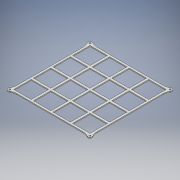
# Autodesk Inventor part: b-base
Saved by Autodesk Inventor 2017 (Build 210142000, 142)
## iProperties
Created: 2019-02-09
Part Number: b-base
Material: Generic
Document SubType Name: Modeling
Designer: felix
Density: 1 g/cm^3
Appearance: Default
Author: felix
Autodesk Inventor part; units mm, degrees
ref_plane "YZ Plane" through (0, 0, 0) normal (1, 0, 0) x (0, 1, 0)
ref_plane "XZ Plane" through (0, 0, 0) normal (0, 1, 0) x (-1, 0, 0)
ref_plane "XY Plane" through (0, 0, 0) normal (0, 0, 1) x (1, 0, 0)
sketch "Sketch1" plane through (0, 0, 0) normal (0, 0, 1) x (1, 0, 0)
  line L0 (-23.6233, -6.7963) -> (65.3767, -6.7963)
  line L1 (65.3767, -6.7963) -> (65.3767, 82.2037)
  line L2 (65.3767, 82.2037) -> (-23.6233, 82.2037)
  line L3 (-23.6233, 82.2037) -> (-23.6233, -6.7963)
  line L4 (-23.6233, 93.2037) -> (65.3767, 93.2037)
  line L5 (65.3767, 93.2037) -> (65.3767, 182.2037)
  line L6 (65.3767, 182.2037) -> (-23.6233, 182.2037)
  line L7 (-23.6233, 182.2037) -> (-23.6233, 93.2037)
  line L8 (-23.6233, 193.2037) -> (65.3767, 193.2037)
  line L9 (65.3767, 193.2037) -> (65.3767, 282.2037)
  line L10 (65.3767, 282.2037) -> (-23.6233, 282.2037)
  line L11 (-23.6233, 282.2037) -> (-23.6233, 193.2037)
  line L12 (-23.6233, 293.2037) -> (65.3767, 293.2037)
  line L13 (65.3767, 293.2037) -> (65.3767, 382.2037)
  line L14 (65.3767, 382.2037) -> (-23.6233, 382.2037)
  line L15 (-23.6233, 382.2037) -> (-23.6233, 293.2037)
  line L16 (76.3767, -6.7963) -> (165.3767, -6.7963)
  line L17 (165.3767, -6.7963) -> (165.3767, 82.2037)
  line L18 (165.3767, 82.2037) -> (76.3767, 82.2037)
  line L19 (76.3767, 82.2037) -> (76.3767, -6.7963)
  line L20 (76.3767, 93.2037) -> (165.3767, 93.2037)
  line L21 (165.3767, 93.2037) -> (165.3767, 182.2037)
  line L22 (165.3767, 182.2037) -> (76.3767, 182.2037)
  line L23 (76.3767, 182.2037) -> (76.3767, 93.2037)
  line L24 (76.3767, 193.2037) -> (165.3767, 193.2037)
  line L25 (165.3767, 193.2037) -> (165.3767, 282.2037)
  line L26 (165.3767, 282.2037) -> (76.3767, 282.2037)
  line L27 (76.3767, 282.2037) -> (76.3767, 193.2037)
  line L28 (76.3767, 293.2037) -> (165.3767, 293.2037)
  line L29 (165.3767, 293.2037) -> (165.3767, 382.2037)
  line L30 (165.3767, 382.2037) -> (76.3767, 382.2037)
  line L31 (76.3767, 382.2037) -> (76.3767, 293.2037)
  line L32 (176.3767, -6.7963) -> (265.3767, -6.7963)
  line L33 (265.3767, -6.7963) -> (265.3767, 82.2037)
  line L34 (265.3767, 82.2037) -> (176.3767, 82.2037)
  line L35 (176.3767, 82.2037) -> (176.3767, -6.7963)
  line L36 (176.3767, 93.2037) -> (265.3767, 93.2037)
  line L37 (265.3767, 93.2037) -> (265.3767, 182.2037)
  line L38 (265.3767, 182.2037) -> (176.3767, 182.2037)
  line L39 (176.3767, 182.2037) -> (176.3767, 93.2037)
  line L40 (176.3767, 193.2037) -> (265.3767, 193.2037)
  line L41 (265.3767, 193.2037) -> (265.3767, 282.2037)
  line L42 (265.3767, 282.2037) -> (176.3767, 282.2037)
  line L43 (176.3767, 282.2037) -> (176.3767, 193.2037)
  line L44 (176.3767, 293.2037) -> (265.3767, 293.2037)
  line L45 (265.3767, 293.2037) -> (265.3767, 382.2037)
  line L46 (265.3767, 382.2037) -> (176.3767, 382.2037)
  line L47 (176.3767, 382.2037) -> (176.3767, 293.2037)
  line L48 (276.3767, -6.7963) -> (365.3767, -6.7963)
  line L49 (365.3767, -6.7963) -> (365.3767, 82.2037)
  line L50 (365.3767, 82.2037) -> (276.3767, 82.2037)
  line L51 (276.3767, 82.2037) -> (276.3767, -6.7963)
  line L52 (276.3767, 93.2037) -> (365.3767, 93.2037)
  line L53 (365.3767, 93.2037) -> (365.3767, 182.2037)
  line L54 (365.3767, 182.2037) -> (276.3767, 182.2037)
  line L55 (276.3767, 182.2037) -> (276.3767, 93.2037)
  line L56 (276.3767, 193.2037) -> (365.3767, 193.2037)
  line L57 (365.3767, 193.2037) -> (365.3767, 282.2037)
  line L58 (365.3767, 282.2037) -> (276.3767, 282.2037)
  line L59 (276.3767, 282.2037) -> (276.3767, 193.2037)
  line L60 (276.3767, 293.2037) -> (365.3767, 293.2037)
  line L61 (365.3767, 293.2037) -> (365.3767, 382.2037)
  line L62 (365.3767, 382.2037) -> (276.3767, 382.2037)
  line L63 (276.3767, 382.2037) -> (276.3767, 293.2037)
  circle A0 centre (-33.6233, -16.7963) radius 4
  arc A1 (-42.1947, -11.6455) -> (-33.6233, 19.2592) centre (-93.6233, 19.2592) ccw
  arc A2 (2.4322, -16.7963) -> (-28.4725, -25.3677) centre (2.4322, -76.7963) ccw
  arc A3 (-42.1947, -11.6455) -> (-28.4725, -25.3677) centre (-33.6233, -16.7963) ccw
  arc A4 (375.3767, 19.2592) -> (383.9481, -11.6455) centre (435.3767, 19.2592) ccw
  circle A5 centre (375.3767, -16.7963) radius 4
  arc A6 (370.2259, -25.3677) -> (383.9481, -11.6455) centre (375.3767, -16.7963) ccw
  arc A7 (370.2259, -25.3677) -> (339.3212, -16.7963) centre (339.3212, -76.7963) ccw
  arc A8 (339.3212, 392.2037) -> (370.2259, 400.7751) centre (339.3212, 452.2037) ccw
  circle A9 centre (375.3767, 392.2037) radius 4
  arc A10 (383.9481, 387.0529) -> (370.2259, 400.7751) centre (375.3767, 392.2037) ccw
  arc A11 (383.9481, 387.0529) -> (375.3767, 356.1482) centre (435.3767, 356.1482) ccw
  arc A12 (-33.6233, 356.1482) -> (-42.1947, 387.0529) centre (-93.6233, 356.1482) ccw
  circle A13 centre (-33.6233, 392.2037) radius 4
  arc A14 (-28.4725, 400.7751) -> (-42.1947, 387.0529) centre (-33.6233, 392.2037) ccw
  arc A15 (-28.4725, 400.7751) -> (2.4322, 392.2037) centre (2.4322, 452.2037) ccw
  line L64 (2.4322, -16.7963) -> (339.3212, -16.7963)
  line L65 (375.3767, 19.2592) -> (375.3767, 356.1482)
  line L66 (-33.6233, 356.1482) -> (-33.6233, 19.2592)
  line L67 (339.3212, 392.2037) -> (2.4322, 392.2037)
  point P0 (0, 0)
  point P1 (0, 100)
  point P2 (0, 200)
  point P3 (0, 300)
  point P4 (100, 0)
  point P5 (100, 100)
  point P6 (100, 200)
  point P7 (100, 300)
  point P8 (200, 0)
  point P9 (200, 100)
  point P10 (200, 200)
  point P11 (200, 300)
  point P12 (300, 0)
  point P13 (300, 100)
  point P14 (300, 200)
  point P15 (300, 300)
  point P16 (170.8767, 187.7037)
  dimension "d0" = 89
  dimension "d1" = 89
  dimension "d4" = 100
  dimension "d7" = 100
  dimension "d10" = 8
  dimension "d11" = 10
  dimension "d12" = 10
  dimension "d17" = 60
  dimension "d18" = 60
  dimension "d21" = 360
  constraints: 136 end point, 24 point on circle, 16 centre point, 4 coincident, 4 parallel, 3 horizontal, 2 collinear, 2 perpendicular, 2 tangent, 1 vertical, 182 other
  measures "d0" distance of L2.end L1.end
  measures "d1" distance of L1.end L0.end
  measures "d4" distance of point (0, 0) point (0, 100)
  measures "d7" distance of point (0, 0) point (100, 0)
  measures "d10" diameter of A0
  measures "d11" distance from line of A0.centre L0
  measures "d12" distance from line of A0.centre L3
  measures "d17" radius of A1
  measures "d18" radius of A2
extrude "Extrusion1" add sketch "Sketch1" along normal blind 5
sketch "Sketch2" plane through (0, 0, 5) normal (0, 0, 1) x (1, 0, 0)
  line L0 (165.3767, 182.2037) -> (165.3767, 93.2037) projected
  line L1 (265.3767, 193.2037) -> (176.3767, 193.2037) projected
  line L2 (165.3767, 182.2037) -> (176.3767, 182.2037)
  line L3 (176.3767, 182.2037) -> (176.3767, 193.2037)
  line L4 (176.3767, 193.2037) -> (165.3767, 193.2037)
  line L5 (165.3767, 193.2037) -> (165.3767, 182.2037)
  point P0 (0, 0)
  point P1 (170.8767, 187.7037)
  constraints: 8 end point, 2 parallel, 1 horizontal, 1 perpendicular
body "Solid1"
